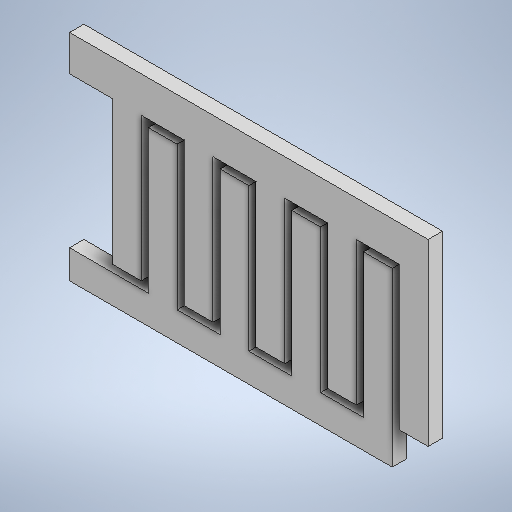
# Autodesk Inventor part: Sensor_0001_001
Saved by Autodesk Inventor 2025.2 (Build 292293000, 293)
## iProperties
Created: 2025-03-19
Part Number: Sensor_0001_001
Material: Genérico
Document SubType Name: Modeling
Designer: lucas
Density: 1 g/cm^3
Appearance: Padrão
Author: lucas
Autodesk Inventor part; units mm, degrees
ref_plane "YZ Plane" through (0, 0, 0) normal (1, 0, 0) x (0, 1, 0)
ref_plane "XZ Plane" through (0, 0, 0) normal (0, 1, 0) x (-1, 0, 0)
ref_plane "XY Plane" through (0, 0, 0) normal (0, 0, 1) x (1, 0, 0)
sketch "Esboço1" plane through (0, 0, 0) normal (0, 0, 1) x (1, 0, 0)
  line L0 (-25, 10) -> (-25, 15)
  line L1 (-25, 15) -> (25, 15)
  line L2 (25, 15) -> (25, -10)
  line L3 (25, -10) -> (21, -10)
  line L4 (21, -10) -> (21, 10)
  line L5 (15, 10) -> (21, 10)
  line L6 (15, 10) -> (15, -10)
  line L7 (1, -10) -> (5, -10)
  line L8 (1, 10) -> (1, -10)
  line L9 (11, -10) -> (15, -10)
  line L10 (11, 10) -> (11, -10)
  line L11 (5, 10) -> (11, 10)
  line L12 (5, 10) -> (5, -10)
  line L13 (-9, 10) -> (-9, -10)
  line L14 (-5, 10) -> (-5, -10)
  line L15 (-5, 10) -> (1, 10)
  line L16 (-9, -10) -> (-5, -10)
  line L17 (-15, 10) -> (-9, 10)
  line L18 (-19, 10) -> (-19, -10)
  line L19 (-15, 10) -> (-15, -10)
  line L20 (-25, 10) -> (-19, 10)
  line L21 (-19, -10) -> (-15, -10)
  line L22 (-25, -15) -> (20, -15)
  line L23 (-25, -11) -> (-25, -15)
  line L24 (-10, -11) -> (-4, -11)
  line L25 (-10, 9) -> (-10, -11)
  line L26 (-14, 9) -> (-14, -11)
  line L27 (6, -11) -> (6, 9)
  line L28 (16, 9) -> (16, -11)
  line L29 (10, 9) -> (10, -11)
  line L30 (-4, 9) -> (-4, -11)
  line L31 (0, 9) -> (0, -11)
  line L32 (20, 9) -> (20, -15)
  line L33 (-25, -11) -> (-14, -11)
  line L34 (-14, 9) -> (-10, 9)
  line L35 (-4, 9) -> (0, 9)
  line L36 (0, -11) -> (6, -11)
  line L37 (6, 9) -> (10, 9)
  line L38 (16, 9) -> (20, 9)
  line L39 (10, -11) -> (16, -11)
  point P0 (0, 0)
  point P1 (0, 15)
  point P2 (-2.5, -15)
  dimension "d5" = 5
  dimension "d6" = 50
  dimension "d7" = 15
  dimension "d9" = 25
  dimension "d10" = 4
  dimension "d12" = 6
  dimension "d37" = 4
  dimension "d39" = 15
  dimension "d43" = 1
  dimension "d45" = 1
  constraints: 80 end point, 26 equal length, 20 vertical, 15 horizontal, 7 horizontal alignment, 4 vertical alignment, 2 midpoint
  measures "d5" distance of L0.end L0.start
  measures "d6" distance of L0.end L1.end
  measures "d7" distance of point (0, 0) point (0, 15)
  measures "d9" distance of L1.end L2.end
  measures "d10" distance of L2.end L3.end
  measures "d12" distance of L5.start L4.end
  measures "d37" distance of L23.start L22.start
  measures "d39" vertical distance of point (-2.5, -15) point (0, 0)
  measures "d43" distance between parallel lines of L19 L26
  measures "d45" distance between parallel lines of L34 L17
extrude "Extrusão1" add sketch "Esboço1" along normal mid plane 2
